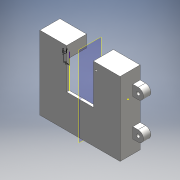
# Autodesk Inventor part: PRING_piston_holder_half
Saved by Autodesk Inventor 2018 (Build 220112000, 112)
## iProperties
Created: 2026-06-13
Part Number: PRING_piston_holder_half
Material: Generic
Document SubType Name: Modeling
Designer: neo
Density: 1 g/cm^3
Appearance: Default
Author: neo
Autodesk Inventor part; units mm, degrees
ref_plane "YZ Plane" through (0, 0, 0) normal (1, 0, 0) x (0, 1, 0)
ref_plane "XZ Plane" through (0, 0, 0) normal (0, 1, 0) x (-1, 0, 0)
ref_plane "XY Plane" through (0, 0, 0) normal (0, 0, 1) x (1, 0, 0)
sketch "Sketch1" plane through (0, 0, 0) normal (0, 1, 0) x (-1, 0, 0)
  circle A0 centre (0, 0) radius 2.5
  circle A1 centre (0, -55) radius 2.5
  arc A2 (0, 8) -> (0, -8) centre (0, 0) ccw
  arc A3 (0, -47) -> (0, -63) centre (0, -55) ccw
  line L0 (0, -63) -> (8, -63)
  line L1 (8, -63) -> (8, -47)
  line L2 (0, -47) -> (8, -47)
  line L3 (0, -8) -> (8, -8)
  line L4 (8, -8) -> (8, 8)
  line L5 (8, 8) -> (0, 8)
  line L6 (0, 2.5) -> (0, -2.5)
  line L7 (0, 0) -> (0, -2.5) construction
  line L8 (0, -8) -> (0, -49.9553) construction
  dimension "d0" = 5
  dimension "d1" = 5
  dimension "d2" = 55
  dimension "d3" = 16
  dimension "d4" = 16
  constraints: 18 end point, 6 point on circle, 4 centre point, 3 coincident, 3 perpendicular, 2 horizontal, 2 parallel, 2 vertical, 1 tangent
  measures "d0" diameter of A0
  measures "d1" diameter of A1
  measures "d2" distance of L7.start A1.centre
  measures "d3" diameter of A2
  measures "d4" diameter of A3
extrude "Extrusion1" add sketch "Sketch1" along normal blind 12.45
sketch "Sketch3" plane through (0, 0, 0) normal (0, -1, 0) x (1, 0, 0)
  circle A0 centre (0, -55) radius 2.5 construction
  arc A1 (0, -63) -> (0, -47) centre (0, -55) ccw construction
  line L0 (0, -47) -> (-8, -47) construction
  line L1 (-8, -47) -> (-8, -63) construction
  line L2 (-8, -63) -> (0, -63) construction
  circle A2 centre (0, 0) radius 2.5 construction
  arc A3 (0, -8) -> (0, 8) centre (0, 0) ccw construction
  line L3 (0, 8) -> (-8, 8) construction
  line L4 (-8, 8) -> (-8, -8) construction
  line L5 (-8, -8) -> (0, -8) construction
  line L6 (-8, -82.5) -> (-68, -82.5)
  line L7 (-68, -82.5) -> (-68, 27.5)
  line L8 (-68, 27.5) -> (-8, 27.5)
  line L9 (-8, 27.5) -> (-8, -82.5)
  line L10 (-68, -27.5) -> (7.195, -27.5) construction
  circle A4 centre (0, 0) radius 2.5 construction
  circle A5 centre (0, -55) radius 2.5 construction
  line L11 (-8, -8) -> (-8, 8) projected
  dimension "d15" = 27.5
  dimension "d16" = 110
  dimension "d22" = 60
  constraints: 10 end point, 2 horizontal, 2 parallel, 1 collinear, 1 midpoint, 1 perpendicular
  measures "d15" distance from line of point (0, 0) L10
  measures "d16" distance of L6.end L7.end
  measures "d22" distance of L7.end L8.end
extrude "Extrusion3" add sketch "Sketch3" along normal blind 17.55 and the other way blind 12.45
sketch "Sketch4" plane through (0, 12.45, 0) normal (0, 1, 0) x (1, 0, 0)
  line L0 (-8, 8) -> (-8, 47) construction
  line L1 (-8, 82.5) -> (-68, 82.5) construction
  line L2 (-68, 82.5) -> (-68, -27.5) construction
  line L3 (-68, -27.5) -> (-8, -27.5) construction
  line L4 (-28, -37.155) -> (-28, 112.7267) construction
  line L5 (-28, -22.5) -> (-30.05, -22.5)
  line L6 (-30.05, -22.5) -> (-30.05, 78.5)
  line L7 (-30.05, 78.5) -> (-28, 78.5)
  line L8 (-28, 78.5) -> (-28, -22.5)
  arc A0 (0, -8) -> (0, 8) centre (0, 0) ccw projected
  line L9 (0, 8) -> (-8, 8) projected
  line L10 (-8, 47) -> (0, 47) projected
  arc A1 (0, 47) -> (0, 63) centre (0, 55) ccw projected
  line L11 (0, 63) -> (-8, 63) projected
  line L12 (-8, 63) -> (-8, 82.5) projected
  line L13 (-8, -27.5) -> (-8, -8) projected
  line L14 (-8, -8) -> (0, -8) projected
  dimension "d17" = 20
  dimension "d18" = 2.05
  dimension "d19" = 101
  dimension "d20" = 5
  constraints: 10 end point, 2 parallel, 1 horizontal, 1 perpendicular, 1 point on line, 1 vertical
  measures "d17" distance between parallel lines of L0 L4
  measures "d18" distance between parallel lines of L4 L6
  measures "d19" distance of L5.end L6.end
  measures "d20" distance between parallel lines of L3 L5
revolve "guide_rail_mount" cut sketch "Sketch4" angle 360 about axis through (-28, 12.45, 37.155) along (0, 0, -1)
mirror "Mirror1" about plane through (-68, 0, 27.5) normal (-1, 0, 0)
sketch "Sketch5" plane through (0, 12.45, 0) normal (0, 1, 0) x (1, 0, 0)
  line L0 (-128, 8) -> (-128, 47) construction
  line L1 (-128, 27.5) -> (-8, 27.5) construction
  line L2 (-8, 82.5) -> (-8, -27.5) construction
  line L3 (-8, -27.5) -> (-128, -27.5) construction
  line L4 (-68, -27.5) -> (-68, 82.5) construction
  line L5 (-123, -17.5) -> (-13, -17.5)
  line L6 (-13, -17.5) -> (-13, 72.5)
  line L7 (-13, 72.5) -> (-123, 72.5)
  line L8 (-123, 72.5) -> (-123, -17.5)
  point P0 (0, 0)
  dimension "d23" = 10
  dimension "d26" = 5
  constraints: 12 end point, 3 midpoint, 2 parallel, 1 horizontal, 1 perpendicular, 1 vertical, 2 other
  measures "d23" distance between parallel lines of L3 L5
  measures "d26" distance between parallel lines of L8 L0
extrude "Extrusion4" cut sketch "Sketch5" against normal blind 26
sketch "Sketch6" plane through (0, 12.45, 0) normal (0, 1, 0) x (1, 0, 0)
  line L0 (-68, -27.5) -> (-68, 79.7854) construction
  line L1 (-88, -32.5) -> (-48, -32.5)
  line L2 (-48, -32.5) -> (-48, 32.5)
  line L3 (-48, 32.5) -> (-88, 32.5)
  line L4 (-88, 32.5) -> (-88, -32.5)
  line L5 (-8, -27.5) -> (-128, -27.5) projected
  line L6 (-105.95, 72.5) -> (-30.05, 72.5) projected
  line L7 (-68, 72.5) -> (-68, 96.7026) construction
  point P0 (0, 0)
  dimension "d27" = 5
  dimension "d28" = 60
  dimension "d29" = 40
  constraints: 12 end point, 2 parallel, 2 vertical, 1 collinear, 1 horizontal, 1 midpoint, 1 perpendicular, 1 other
  measures "d27" distance between parallel lines of L1 L5
  measures "d28" distance between parallel lines of L5 L3
  measures "d29" distance of L1.start L1.end
extrude "Extrusion5" cut sketch "Sketch6" against normal through all
sketch "Sketch7" plane through (0, -13.55, 0) normal (0, 1, 0) x (1, 0, 0)
  line L0 (-88, -17.5) -> (-88, 32.5) projected
  line L1 (-88, -17.5) -> (-96, -17.5)
  line L2 (-96, -17.5) -> (-96, -9.5)
  line L3 (-96, -9.5) -> (-88, -9.5)
  line L4 (-88, -9.5) -> (-88, -17.5)
  line L5 (-88, -17.5) -> (-105.95, -17.5) projected
  circle A0 centre (-92, -17.5) radius 1.5
  point P0 (0, 0)
  dimension "d32" = 8
  dimension "d33" = 8
  dimension "d36" = 3
  constraints: 8 end point, 2 parallel, 1 centre point, 1 horizontal, 1 perpendicular, 1 point on line
  measures "d32" distance of L1.end L2.end
  measures "d33" distance of L2.end L3.end
  measures "d36" diameter of A0
extrude "Extrusion6" add sketch "Sketch7" along normal blind 26 contours L1 A0 L2 L3 L0 | L1 A0 picked at (-91.8227, -17.0325)
ref_plane "Work Plane1" through (-68, -17.55, -82.5) normal (-1, 0, 0) x (0, 0, 1)
extrude "Extrusion7" cut sketch "Sketch7" along normal through all both and the other way through all contours A0 L1 | L1 A0
mirror "Mirror2" about plane through (-68, -17.55, -82.5) normal (-1, 0, 0) of "Extrusion6", "Extrusion7"
sketch "Sketch8" plane through (0, 12.45, 0) normal (0, 1, 0) x (1, 0, 0)
  line L0 (-98, 65.1826) -> (-38, 65.1826)
  line L1 (-38, 65.1826) -> (-38, 77.5)
  line L2 (-38, 77.5) -> (-98, 77.5)
  line L3 (-98, 77.5) -> (-98, 65.1826)
  line L4 (-68, -49.5) -> (-68, 104.5) construction
  line L5 (-105.95, 72.5) -> (-30.05, 72.5) construction
  point P0 (0, 0)
  dimension "d39" = 60
  dimension "d40" = 5
  constraints: 8 end point, 2 parallel, 1 horizontal, 1 perpendicular, 1 other
  measures "d39" distance between parallel lines of L1 L3
  measures "d40" distance between parallel lines of L5 L2
extrude "Extrusion8" cut sketch "Sketch8" against normal blind 18
sketch "Sketch9" plane through (0, 0, 8) normal (0, 0, 1) x (1, 0, 0)
  line L0 (0, 0) -> (-8, 0) construction
  line L1 (0, 0) -> (0, 12.45) construction
  line L2 (-8, 12.45) -> (0, 12.45) construction
  line L3 (-8, 0) -> (-8, 12.45) construction
  line L4 (-8, 0) -> (-8, 12.45) projected
  line L5 (-8, 1.45) -> (23.9687, 1.45)
  line L6 (23.9687, 1.45) -> (23.9687, -24.0835)
  line L7 (23.9687, -24.0835) -> (-8, -24.0835)
  line L8 (-8, -24.0835) -> (-8, 1.45)
  point P0 (0, 0)
  dimension "d43" = 11
  constraints: 8 end point, 2 parallel, 1 horizontal, 1 perpendicular, 1 point on line
  measures "d43" distance between parallel lines of L2 L5
extrude "limit-side-to-11mm" cut sketch "Sketch9" against normal through all
mirror "Mirror3" about plane through (-68, -17.55, -82.5) normal (-1, 0, 0) of "limit-side-to-11mm"
equation "\"d15\" = 0.25 * d16"
body "Solid1"
